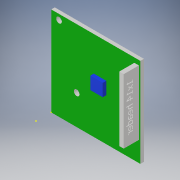
# Autodesk Inventor part: Part1
Saved by Autodesk Inventor 2017 (Build 210142000, 142)
## iProperties
Created: 2016-10-27
Part Number: Part1
Material: Generic
Document SubType Name: Modeling
Designer: cad
Density: 1 g/cm^3
Appearance: Default
Author: cad
Autodesk Inventor part; units mm, degrees
ref_plane "YZ Plane" through (0, 0, 0) normal (1, 0, 0) x (0, 1, 0)
ref_plane "XZ Plane" through (0, 0, 0) normal (0, 1, 0) x (-1, 0, 0)
ref_plane "XY Plane" through (0, 0, 0) normal (0, 0, 1) x (1, 0, 0)
sketch "Sketch1" plane through (0, 0, 0) normal (0, 0, 1) x (1, 0, 0)
  point P0 (0, 0)
sketch "Sketch2" plane through (0, 0, 0) normal (0, 0, 1) x (1, 0, 0)
  line L0 (0, 0) -> (50, 0)
  line L1 (50, 0) -> (50, 50)
  line L2 (50, 50) -> (0, 50)
  circle A0 centre (4.4, 47) radius 1.6
  circle A1 centre (14.3, 16.7) radius 1.6
  line L3 (0, 50) -> (3, 50) construction
  circle A2 centre (41.9, 12.5) radius 1.6
  line L4 (30.9, 23.8) -> (30.9, 30.8)
  line L5 (30.9, 30.8) -> (23.9, 30.8)
  line L6 (23.9, 30.8) -> (23.9, 23.8)
  line L7 (23.9, 23.8) -> (30.9, 23.8)
  line L8 (0, 50) -> (0, 0)
  dimension "d0" = 50
  dimension "d1" = 50
  dimension "d2" = 3.2
  dimension "d3" = 3.2
  dimension "d23" = 3.2
  dimension "d28" = 7
  dimension "d29" = 7
  dimension "d30" = 7
  dimension "d31" = 90
  constraints: 18 end point, 3 centre point, 3 horizontal, 3 perpendicular, 1 parallel, 1 vertical
  measures "d0" distance of L2.end L1.end
  measures "d1" distance of L1.end L0.end
  measures "d2" diameter of A0
  measures "d3" diameter of A1
  measures "d23" diameter of A2
  measures "d28" distance of L4.start L4.end
  measures "d29" distance of L4.end L5.end
  measures "d30" distance of L5.end L6.end
  measures "d31" angle of L6 L5
sketch "Sketch7" plane through (0, 0, 0) normal (0, 0, 1) x (1, 0, 0)
  line L0 (30.9, 23.8) -> (30.9, 30.8)
  line L1 (30.9, 30.8) -> (23.9, 30.8)
  line L2 (23.9, 30.8) -> (23.9, 23.8)
  line L3 (23.9, 23.8) -> (30.9, 23.8)
  point P0 (0, 0)
  dimension "d32" = 7
  dimension "d33" = 7
  dimension "d34" = 7
  dimension "d35" = 90
  constraints: 8 end point, 2 perpendicular, 1 horizontal
  measures "d32" distance of L0.start L1.start
  measures "d33" distance of L1.start L1.end
  measures "d34" distance of L1.end L3.start
  measures "d35" angle of L2 L1
extrude "Extrusion4" add sketch "Sketch2" against normal blind 2 contours L8 L2 L1 L0 | L7 L6 L5 L4
extrude "Extrusion5" add sketch "Sketch7" along normal blind 2 separate body
sketch "Sketch8" plane through (0, 0, 0) normal (0, 0, 1) x (1, 0, 0)
  line L0 (46.63, 47.4) -> (46.63, 11.24)
  line L1 (46.63, 11.24) -> (49.17, 11.24)
  line L2 (49.17, 11.24) -> (49.17, 47.4)
  line L3 (46.63, 47.4) -> (49.17, 47.4)
  point P0 (0, 0)
  constraints: 8 end point, 1 horizontal, 1 perpendicular
extrude "Extrusion6" add sketch "Sketch8" along normal blind 8.5 separate body
sketch "Sketch9" plane through (0, 0, 8.5) normal (0, 0, 1) x (1, 0, 0)
  point P0 (0, 0)
sketch "Sketch14" plane through (46.63, 11.24, 0) normal (-1, 0, 0) x (0, 0, 1)
  line L0 (7.006, 31.5781) -> (7.006, -2.6918) construction
  line L1 (7.006, -2.6918) -> (-19.1418, -2.6918) construction
  line L2 (-19.1418, -2.6918) -> (-19.1418, 31.5781) construction
  line L3 (-19.1418, 31.5781) -> (7.006, 31.5781) construction
  line L4 (3.35, 29.3402) -> (3.35, 31.0477)
  line L5 (3.35, 31.0477) -> (3.7074, 31.0477)
  line L6 (3.7074, 31.0477) -> (3.7074, 30.4124)
  line L7 (3.7074, 30.4124) -> (6.053, 30.4124)
  line L8 (6.053, 30.4124) -> (6.053, 31.0477)
  line L9 (6.053, 31.0477) -> (6.3735, 31.0477)
  spline S0 degree 2 poles (6.3735, 31.0477) (6.3735, 30.6875) (6.5777, 30.3471) (6.8614, 30.3244) knots 0 0 0 1 2 2 2
  line L10 (6.8614, 30.3244) -> (6.8614, 29.9614)
  line L11 (6.8614, 29.9614) -> (3.7074, 29.9614)
  line L12 (3.7074, 29.9614) -> (3.7074, 29.3402)
  line L13 (3.7074, 29.3402) -> (3.35, 29.3402)
  line L14 (3.35, 26.5919) -> (3.35, 27.1336)
  line L15 (3.35, 27.1336) -> (4.3371, 27.7718)
  line L16 (4.3371, 27.7718) -> (3.35, 28.427)
  line L17 (3.35, 28.427) -> (3.35, 28.929)
  line L18 (3.35, 28.929) -> (4.6519, 28.0185)
  line L19 (4.6519, 28.0185) -> (5.9765, 28.9205)
  line L20 (5.9765, 28.9205) -> (5.9765, 28.3787)
  line L21 (5.9765, 28.3787) -> (4.9979, 27.7434)
  line L22 (4.9979, 27.7434) -> (5.9765, 27.0939)
  line L23 (5.9765, 27.0939) -> (5.9765, 26.5919)
  line L24 (5.9765, 26.5919) -> (4.6803, 27.4966)
  line L25 (4.6803, 27.4966) -> (3.35, 26.5919)
  line L26 (3.35, 24.3313) -> (3.35, 26.0388)
  line L27 (3.35, 26.0388) -> (3.7074, 26.0388)
  line L28 (3.7074, 26.0388) -> (3.7074, 25.4035)
  line L29 (3.7074, 25.4035) -> (6.053, 25.4035)
  line L30 (6.053, 25.4035) -> (6.053, 26.0388)
  line L31 (6.053, 26.0388) -> (6.3735, 26.0388)
  spline S1 degree 2 poles (6.3735, 26.0388) (6.3735, 25.6786) (6.5777, 25.3382) (6.8614, 25.3155) knots 0 0 0 1 2 2 2
  line L32 (6.8614, 25.3155) -> (6.8614, 24.9525)
  line L33 (6.8614, 24.9525) -> (3.7074, 24.9525)
  line L34 (3.7074, 24.9525) -> (3.7074, 24.3313)
  line L35 (3.7074, 24.3313) -> (3.35, 24.3313)
  line L36 (4.5526, 21.4355) -> (4.5526, 21.8524)
  line L37 (4.5526, 21.8524) -> (3.35, 21.8524)
  line L38 (3.35, 21.8524) -> (3.35, 22.3034)
  line L39 (3.35, 22.3034) -> (4.5526, 22.3034)
  line L40 (4.5526, 22.3034) -> (4.5526, 23.8492)
  line L41 (4.5526, 23.8492) -> (5.0461, 23.8492)
  line L42 (5.0461, 23.8492) -> (6.85, 22.2835)
  line L43 (6.85, 22.2835) -> (6.85, 21.8524)
  line L44 (6.85, 21.8524) -> (4.9299, 21.8524)
  line L45 (4.9299, 21.8524) -> (4.9299, 21.4355)
  line L46 (4.9299, 21.4355) -> (4.5526, 21.4355)
  line L47 (4.9299, 22.3034) -> (6.297, 22.3034)
  line L48 (6.297, 22.3034) -> (4.9299, 23.4804)
  line L49 (4.9299, 23.4804) -> (4.9299, 22.3034)
  line L50 (3.35, 17.4306) -> (3.35, 17.8731)
  line L51 (3.35, 17.8731) -> (4.8476, 17.8731)
  spline S2 degree 2 poles (4.8476, 17.8731) (5.0291, 17.8731) (5.3411, 17.9071) (5.4347, 17.9582) knots 0 0 0 1 2 2 2
  spline S3 degree 2 poles (5.4347, 17.9582) (5.534, 18.012) (5.6304, 18.2049) (5.6304, 18.3694) knots 0 0 0 1 2 2 2
  spline S4 degree 2 poles (5.6304, 18.3694) (5.6304, 18.5339) (5.4546, 18.8828) (5.3128, 19.0501) knots 0 0 0 1 2 2 2
  line L52 (5.3128, 19.0501) -> (3.35, 19.0501)
  line L53 (3.35, 19.0501) -> (3.35, 19.4926)
  line L54 (3.35, 19.4926) -> (7.006, 19.4926)
  line L55 (7.006, 19.4926) -> (7.006, 19.0501)
  line L56 (7.006, 19.0501) -> (5.6843, 19.0501)
  spline S5 degree 2 poles (5.6843, 19.0501) (5.863, 18.8516) (6.0502, 18.4687) (6.0502, 18.2531) knots 0 0 0 1 2 2 2
  spline S6 degree 2 poles (6.0502, 18.2531) (6.0502, 17.8674) (5.5397, 17.4306) (5.0547, 17.4306) knots 0 0 0 1 2 2 2
  line L57 (5.0547, 17.4306) -> (3.35, 17.4306)
  spline S7 degree 2 poles (3.2905, 15.6693) (3.2905, 16.2989) (3.9967, 16.991) (4.6491, 16.991) knots 0 0 0 1 2 2 2
  spline S8 degree 2 poles (4.6491, 16.991) (5.2901, 16.991) (6.0502, 16.3188) (6.0502, 15.777) knots 0 0 0 1 2 2 2
  spline S9 degree 2 poles (6.0502, 15.777) (6.0502, 15.5331) (5.9084, 15.1559) (5.7581, 15.0169) knots 0 0 0 1 2 2 2
  spline S10 degree 2 poles (5.7581, 15.0169) (5.6077, 14.8751) (5.1738, 14.7248) (4.8589, 14.7248) knots 0 0 0 1 2 2 2
  line L58 (4.8589, 14.7248) -> (4.6179, 14.7248)
  line L59 (4.6179, 14.7248) -> (4.6179, 16.5428)
  spline S11 degree 2 poles (4.6179, 16.5428) (4.1612, 16.5428) (3.6762, 16.0834) (3.6762, 15.6749) knots 0 0 0 1 2 2 2
  spline S12 degree 2 poles (3.6762, 15.6749) (3.6762, 15.5303) (3.7414, 15.2495) (3.7925, 15.136) knots 0 0 0 1 2 2 2
  spline S13 degree 2 poles (3.7925, 15.136) (3.8492, 15.0169) (3.9485, 14.8524) (3.9939, 14.7985) knots 0 0 0 1 2 2 2
  line L60 (3.9939, 14.7985) -> (3.9939, 14.773)
  line L61 (3.9939, 14.773) -> (3.5117, 14.773)
  spline S14 degree 2 poles (3.5117, 14.773) (3.4805, 14.8496) (3.3897, 15.0821) (3.3642, 15.1729) knots 0 0 0 1 2 2 2
  spline S15 degree 2 poles (3.3642, 15.1729) (3.3273, 15.3005) (3.2905, 15.5104) (3.2905, 15.6693) knots 0 0 0 1 2 2 2
  spline S16 degree 2 poles (4.9554, 15.1559) (5.1341, 15.1616) (5.395, 15.2353) (5.4829, 15.3062) knots 0 0 0 1 2 2 2
  spline S17 degree 2 poles (5.4829, 15.3062) (5.5822, 15.3828) (5.6871, 15.6239) (5.6871, 15.8026) knots 0 0 0 1 2 2 2
  spline S18 degree 2 poles (5.6871, 15.8026) (5.6871, 15.9784) (5.5822, 16.2252) (5.4801, 16.3273) knots 0 0 0 1 2 2 2
  spline S19 degree 2 poles (5.4801, 16.3273) (5.3752, 16.4265) (5.1227, 16.5287) (4.9554, 16.5428) knots 0 0 0 1 2 2 2
  line L62 (4.9554, 16.5428) -> (4.9554, 15.1559)
  spline S20 degree 2 poles (3.628, 12.8131) (3.5883, 12.867) (3.4465, 13.0485) (3.4039, 13.1336) knots 0 0 0 1 2 2 2
  spline S21 degree 2 poles (3.4039, 13.1336) (3.3415, 13.2499) (3.2763, 13.4683) (3.2763, 13.6668) knots 0 0 0 1 2 2 2
  spline S22 degree 2 poles (3.2763, 13.6668) (3.2763, 13.8285) (3.3983, 14.1206) (3.5089, 14.2312) knots 0 0 0 1 2 2 2
  spline S23 degree 2 poles (3.5089, 14.2312) (3.6166, 14.3362) (3.9343, 14.4638) (4.1102, 14.4638) knots 0 0 0 1 2 2 2
  spline S24 degree 2 poles (4.1102, 14.4638) (4.3824, 14.4638) (4.7682, 14.2341) (4.8788, 13.9845) knots 0 0 0 1 2 2 2
  spline S25 degree 2 poles (4.8788, 13.9845) (4.9809, 13.7633) (5.0575, 13.162) (5.0773, 12.8131) knots 0 0 0 1 2 2 2
  line L63 (5.0773, 12.8131) -> (5.1624, 12.8131)
  spline S26 degree 2 poles (5.1624, 12.8131) (5.3156, 12.8131) (5.5056, 12.9067) (5.5595, 12.9918) knots 0 0 0 1 2 2 2
  spline S27 degree 2 poles (5.5595, 12.9918) (5.6134, 13.0769) (5.6474, 13.3208) (5.6474, 13.4513) knots 0 0 0 1 2 2 2
  spline S28 degree 2 poles (5.6474, 13.4513) (5.6474, 13.6044) (5.5567, 14.0185) (5.4688, 14.2256) knots 0 0 0 1 2 2 2
  line L64 (5.4688, 14.2256) -> (5.4688, 14.2511)
  line L65 (5.4688, 14.2511) -> (5.9197, 14.2511)
  spline S29 degree 2 poles (5.9197, 14.2511) (5.9538, 14.1291) (6.0389, 13.6725) (6.0389, 13.4484) knots 0 0 0 1 2 2 2
  spline S30 degree 2 poles (6.0389, 13.4484) (6.0389, 13.1761) (5.9538, 12.8046) (5.8431, 12.6571) knots 0 0 0 1 2 2 2
  spline S31 degree 2 poles (5.8431, 12.6571) (5.7354, 12.5124) (5.3922, 12.3706) (5.1454, 12.3706) knots 0 0 0 1 2 2 2
  line L66 (5.1454, 12.3706) -> (3.35, 12.3706)
  line L67 (3.35, 12.3706) -> (3.35, 12.8131)
  line L68 (3.35, 12.8131) -> (3.628, 12.8131)
  line L69 (3.9967, 12.8131) -> (4.7256, 12.8131)
  spline S32 degree 2 poles (4.7256, 12.8131) (4.7115, 12.9719) (4.6632, 13.4513) (4.6179, 13.6016) knots 0 0 0 1 2 2 2
  spline S33 degree 2 poles (4.6179, 13.6016) (4.564, 13.7774) (4.3399, 14.0072) (4.1414, 14.0072) knots 0 0 0 1 2 2 2
  spline S34 degree 2 poles (4.1414, 14.0072) (3.9145, 14.0072) (3.6847, 13.7519) (3.6847, 13.508) knots 0 0 0 1 2 2 2
  spline S35 degree 2 poles (3.6847, 13.508) (3.6847, 13.3009) (3.8634, 12.9606) (3.9967, 12.8131) knots 0 0 0 1 2 2 2
  line L70 (3.35, 9.73) -> (3.35, 10.1725)
  line L71 (3.35, 10.1725) -> (3.6166, 10.1725)
  spline S36 degree 2 poles (3.6166, 10.1725) (3.5316, 10.2746) (3.4181, 10.4249) (3.3699, 10.527) knots 0 0 0 1 2 2 2
  spline S37 degree 2 poles (3.3699, 10.527) (3.3245, 10.6206) (3.2763, 10.822) (3.2763, 10.9553) knots 0 0 0 1 2 2 2
  spline S38 degree 2 poles (3.2763, 10.9553) (3.2763, 11.1709) (3.455, 11.5339) (3.628, 11.6616) knots 0 0 0 1 2 2 2
  spline S39 degree 2 poles (3.628, 11.6616) (3.801, 11.7892) (4.3115, 11.931) (4.6434, 11.931) knots 0 0 0 1 2 2 2
  spline S40 degree 2 poles (4.6434, 11.931) (4.9894, 11.931) (5.4943, 11.7523) (5.6843, 11.5963) knots 0 0 0 1 2 2 2
  spline S41 degree 2 poles (5.6843, 11.5963) (5.8545, 11.4517) (6.0502, 11.0461) (6.0502, 10.822) knots 0 0 0 1 2 2 2
  spline S42 degree 2 poles (6.0502, 10.822) (6.0502, 10.6263) (5.9623, 10.3342) (5.8715, 10.1725) knots 0 0 0 1 2 2 2
  line L72 (5.8715, 10.1725) -> (7.006, 10.1725)
  line L73 (7.006, 10.1725) -> (7.006, 9.73)
  line L74 (7.006, 9.73) -> (3.35, 9.73)
  line L75 (3.9882, 10.1725) -> (5.5056, 10.1725)
  spline S43 degree 2 poles (5.5056, 10.1725) (5.585, 10.337) (5.6446, 10.5979) (5.6446, 10.7483) knots 0 0 0 1 2 2 2
  spline S44 degree 2 poles (5.6446, 10.7483) (5.6446, 11.0886) (5.1341, 11.4744) (4.6519, 11.4744) knots 0 0 0 1 2 2 2
  spline S45 degree 2 poles (4.6519, 11.4744) (4.1867, 11.4744) (3.6961, 11.1794) (3.6961, 10.8532) knots 0 0 0 1 2 2 2
  spline S46 degree 2 poles (3.6961, 10.8532) (3.6961, 10.6802) (3.8549, 10.3285) (3.9882, 10.1725) knots 0 0 0 1 2 2 2
  spline S47 degree 2 poles (3.2905, 7.9488) (3.2905, 8.5785) (3.9967, 9.2706) (4.6491, 9.2706) knots 0 0 0 1 2 2 2
  spline S48 degree 2 poles (4.6491, 9.2706) (5.2901, 9.2706) (6.0502, 8.5983) (6.0502, 8.0566) knots 0 0 0 1 2 2 2
  spline S49 degree 2 poles (6.0502, 8.0566) (6.0502, 7.8127) (5.9084, 7.4355) (5.7581, 7.2965) knots 0 0 0 1 2 2 2
  spline S50 degree 2 poles (5.7581, 7.2965) (5.6077, 7.1547) (5.1738, 7.0043) (4.8589, 7.0043) knots 0 0 0 1 2 2 2
  line L76 (4.8589, 7.0043) -> (4.6179, 7.0043)
  line L77 (4.6179, 7.0043) -> (4.6179, 8.8224)
  spline S51 degree 2 poles (4.6179, 8.8224) (4.1612, 8.8224) (3.6762, 8.3629) (3.6762, 7.9545) knots 0 0 0 1 2 2 2
  spline S52 degree 2 poles (3.6762, 7.9545) (3.6762, 7.8099) (3.7414, 7.5291) (3.7925, 7.4156) knots 0 0 0 1 2 2 2
  spline S53 degree 2 poles (3.7925, 7.4156) (3.8492, 7.2965) (3.9485, 7.132) (3.9939, 7.0781) knots 0 0 0 1 2 2 2
  line L78 (3.9939, 7.0781) -> (3.9939, 7.0526)
  line L79 (3.9939, 7.0526) -> (3.5117, 7.0526)
  spline S54 degree 2 poles (3.5117, 7.0526) (3.4805, 7.1291) (3.3897, 7.3617) (3.3642, 7.4525) knots 0 0 0 1 2 2 2
  spline S55 degree 2 poles (3.3642, 7.4525) (3.3273, 7.5801) (3.2905, 7.79) (3.2905, 7.9488) knots 0 0 0 1 2 2 2
  spline S56 degree 2 poles (4.9554, 7.4355) (5.1341, 7.4411) (5.395, 7.5149) (5.4829, 7.5858) knots 0 0 0 1 2 2 2
  spline S57 degree 2 poles (5.4829, 7.5858) (5.5822, 7.6624) (5.6871, 7.9035) (5.6871, 8.0821) knots 0 0 0 1 2 2 2
  spline S58 degree 2 poles (5.6871, 8.0821) (5.6871, 8.258) (5.5822, 8.5048) (5.4801, 8.6069) knots 0 0 0 1 2 2 2
  spline S59 degree 2 poles (5.4801, 8.6069) (5.3752, 8.7061) (5.1227, 8.8082) (4.9554, 8.8224) knots 0 0 0 1 2 2 2
  line L80 (4.9554, 8.8224) -> (4.9554, 7.4355)
  line L81 (5.5028, 5.1636) -> (5.5028, 5.1863)
  spline S60 degree 2 poles (5.5028, 5.1863) (5.517, 5.2373) (5.5226, 5.3479) (5.5226, 5.4245) knots 0 0 0 1 2 2 2
  spline S61 degree 2 poles (5.5226, 5.4245) (5.5226, 5.6032) (5.3666, 5.9549) (5.2135, 6.1137) knots 0 0 0 1 2 2 2
  line L82 (5.2135, 6.1137) -> (3.35, 6.1137)
  line L83 (3.35, 6.1137) -> (3.35, 6.5562)
  line L84 (3.35, 6.5562) -> (5.9765, 6.5562)
  line L85 (5.9765, 6.5562) -> (5.9765, 6.1137)
  line L86 (5.9765, 6.1137) -> (5.585, 6.1137)
  spline S62 degree 2 poles (5.585, 6.1137) (5.8006, 5.8727) (5.9765, 5.5124) (5.9765, 5.3423) knots 0 0 0 1 2 2 2
  spline S63 degree 2 poles (5.9765, 5.3423) (5.9765, 5.2742) (5.9708, 5.2061) (5.9623, 5.1636) knots 0 0 0 1 2 2 2
  line L87 (5.9623, 5.1636) -> (5.5028, 5.1636)
  point P0 (0, -11.24)
  constraints: 2 other
extrude "Extrusion7" cut sketch "Sketch14" against normal blind 10 bodies 3
body "Solid2"
body "Solid3"
body "Solid4"
